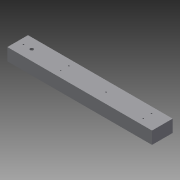
# Autodesk Inventor part: licht_200_support
Saved by Autodesk Inventor 2015 (Build 190159000, 159)
## iProperties
Created: 2018-01-11
Part Number: licht_200_support
Material: Generisch
Document SubType Name: Modeling
Designer: schueler
Density: 1 g/cm^3
Appearance: Vorgabe
Author: schueler
Autodesk Inventor part; units mm, degrees
ref_plane "YZ Plane" through (0, 0, 0) normal (1, 0, 0) x (0, 1, 0)
ref_plane "XZ Plane" through (0, 0, 0) normal (0, 1, 0) x (-1, 0, 0)
ref_plane "XY Plane" through (0, 0, 0) normal (0, 0, 1) x (1, 0, 0)
sketch "Skizze1" plane through (0, 0, 0) normal (0, 0, 1) x (1, 0, 0)
  line L0 (0, 0) -> (350, 0)
  line L1 (350, 50) -> (0, 50)
  line L2 (34, 50) -> (34, 0) construction
  circle A0 centre (34, 25) radius 4
  line L3 (0, 25) -> (350, 25) construction
  circle A1 centre (14, 25) radius 1.5
  circle A2 centre (114, 35) radius 1.5
  circle A3 centre (114, 15) radius 1.5
  circle A4 centre (214, 25) radius 1.5
  circle A5 centre (314, 35) radius 1.5
  circle A6 centre (314, 15) radius 1.5
  line L4 (114, 35) -> (314, 35) construction
  line L5 (314, 35) -> (314, 15) construction
  line L6 (314, 15) -> (114, 15) construction
  line L7 (114, 15) -> (114, 35) construction
  line L8 (0, 50) -> (0, 0)
  line L9 (350, 0) -> (350, 50)
  dimension "d0" = 350
  dimension "d16" = 34
  dimension "d17" = 8
  dimension "d151" = 350
  dimension "d152" = 3
  dimension "d153" = 3
  dimension "d154" = 3
  dimension "d155" = 3
  dimension "d156" = 3
  dimension "d157" = 3
  dimension "d159" = 100
  dimension "d160" = 100
  dimension "d161" = 100
  dimension "d162" = 10
  dimension "d163" = 10
  dimension "d206" = 14
  dimension "d207" = 50
  constraints: 20 end point, 7 centre point, 4 coincident, 4 parallel, 4 point on line, 3 horizontal, 2 midpoint, 2 perpendicular, 1 vertical
  measures "d0" distance of L1.end L1.start
  measures "d16" distance of L1.end L2.start
  measures "d17" diameter of A0
  measures "d151" distance of L3.start L3.end
  measures "d152" diameter of A1
  measures "d153" diameter of A2
  measures "d154" diameter of A3
  measures "d155" diameter of A4
  measures "d156" diameter of A5
  measures "d157" diameter of A6
  measures "d159" distance from line of L7 A1.centre
  measures "d160" distance from line of A4.centre L7
  measures "d161" distance from line of L5 A4.centre
  measures "d162" distance between parallel lines of L3 L4
  measures "d163" distance between parallel lines of L6 L3
  measures "d206" distance from line of L8 A1.centre
  measures "d207" distance of L1.end L0.start
extrude "Extrusion1" add sketch "Skizze1" along normal blind 30
sketch "Skizze6" plane through (0, 50, 0) normal (-1, 0, 0) x (0, 0, 1)
  line L0 (0, -50) -> (30, -50) construction
  line L1 (30, -50) -> (30, 0) construction
  line L2 (30, 0) -> (0, 0) construction
  line L3 (0, 0) -> (0, -50) construction
  line L4 (15, 0) -> (15, -50) construction
  line L5 (0, -29) -> (0, -21) construction
  line L6 (0, -25) -> (30, -25) construction
  point P0 (15, -15)
  point P1 (15, -35)
  dimension "d215" = 10
  dimension "d216" = 10
  constraints: 12 end point, 4 midpoint, 2 parallel, 2 point on line, 1 horizontal, 1 perpendicular
  measures "d215" distance from line of L6 point (15, -15)
  measures "d216" distance from line of L6 point (15, -35)
hole "Bohrung18" at (0, 35, 15) at (0, 15, 15) direction (1, 0, 0) diameter 3 depth 30 tip angle 118
